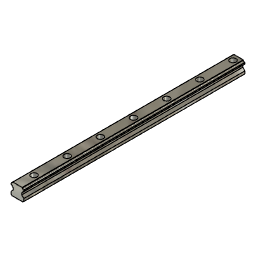
HGR25R_400 (Autodesk Fusion 360 design; units mm, degrees)
Autodesk Fusion 360 part; units mm, degrees
sketch "Sketch2" plane through (0, 0, 0) normal (0, 1, 0) x (1, 0, 0)
  line L0 (0, 0) -> (-10, 0)
  line L1 (-10, 0) -> (-11.5, -1.5)
  line L2 (-11.5, -1.5) -> (-11.5, -6.199)
  line L3 (-11.5, -6.199) -> (-7.7, -9.999)
  line L4 (-7.7, -9.999) -> (-7.7, -13.38)
  line L5 (-11.5, -17.08) -> (-11.5, -19.109)
  line L6 (-8.5085, -22) -> (0, -22)
  line L7 (0, -37) -> (0, 7) construction
  arc A0 (-8.9292, -21.5934) -> (-11.2845, -19.3172) centre (-11.447, -21.842) ccw
  line L8 (-11.5, -19.109) -> (-11.2845, -19.3172)
  line L9 (-8.9292, -21.5934) -> (-8.5085, -22)
  arc A1 (-11.2972, -16.8826) -> (-8.9263, -14.5741) centre (-11.447, -14.357) ccw
  line L10 (-7.7, -13.38) -> (-8.9263, -14.5741)
  line L11 (-11.2972, -16.8826) -> (-11.5, -17.08)
  line L12 (0, 0) -> (10, 0)
  line L13 (10, 0) -> (11.5, -1.5)
  line L14 (11.5, -1.5) -> (11.5, -6.199)
  line L15 (11.5, -6.199) -> (7.7, -9.999)
  line L16 (7.7, -9.999) -> (7.7, -13.38)
  line L17 (7.7, -13.38) -> (8.9263, -14.5741)
  arc A2 (8.9263, -14.5741) -> (11.2972, -16.8826) centre (11.447, -14.357) ccw
  line L18 (11.2972, -16.8826) -> (11.5, -17.08)
  line L19 (11.5, -17.08) -> (11.5, -19.109)
  line L20 (11.5, -19.109) -> (11.2845, -19.3172)
  arc A3 (11.2845, -19.3172) -> (8.9292, -21.5934) centre (11.447, -21.842) ccw
  line L21 (8.9292, -21.5934) -> (8.5085, -22)
  line L22 (8.5085, -22) -> (0, -22)
  dimension "d29" = 10
  dimension "d30" = 1.5
  dimension "d31" = 1.5
  dimension "d32" = 3.381
  dimension "d33" = 3.7
  dimension "d34" = 22
  dimension "d35" = 3.8
  dimension "d36" = 3.8
  dimension "d38" = 8.5085
  dimension "d39" = 2.029
  dimension "d40" = 2.891
  dimension "d42" = 11.447
  dimension "d43" = 0.158
  dimension "d46" = 2.53
  dimension "d47" = 2.53
  dimension "d48" = 7.485
  constraint coincident L0.start L12.start
  constraint horizontal L0
  constraint perpendicular L0 L2
  constraint perpendicular L0 L4
  constraint perpendicular L0 L5
  constraint perpendicular L5 L6
  constraint vertical L7
  constraint collinear L2 L5
  constraint coincident L0.start L7
  constraint coincident L6.end L7
  constraint coincident A0.start L8
  constraint collinear L8 L9
  constraint coincident A1.start L10
  constraint collinear L10 L11
  constraint vertical A0.centre A1.centre
  constraint symmetric L0.start L7 L12.start
  constraint symmetric L0.end L7 L12.end
  constraint symmetric L1.end L7 L13.end
  constraint symmetric L2.end L7 L14.end
  constraint symmetric L3.end L7 L15.end
  constraint symmetric L4.end L7 L16.end
  constraint symmetric L5.start L7 L18.end
  constraint symmetric L5.end L7 L19.end
  constraint symmetric L6.start L7 L21.end
  constraint symmetric L6.end L7 L22.end
  constraint symmetric L7 A0.end L20.end
  constraint symmetric L7 A0.start A3.end
  constraint symmetric L7 A0 A3
  constraint symmetric L7 A1.end L17.end
  constraint symmetric L7 A1.start A2.end
  constraint symmetric L7 A1 A2
  measures "d29" distance of L0.start L0.end
  measures "d30" vertical distance of L0.start L1.end
  measures "d31" distance of L0.end L2
  measures "d32" distance of L3.end L4.end
  measures "d33" vertical distance of L4.end L5.start
  measures "d34" distance of L0.start L6
  measures "d35" vertical distance of L2.end L3.end
  measures "d36" horizontal distance of L2.end L3.end
  measures "d38" distance of L6.start L7
  measures "d39" distance of L5.start L5.end
  measures "d40" distance of L5.end L6
  measures "d42" distance of L7 A0.centre
  measures "d43" distance of L6 A0.centre
  measures "d46" radius of A0
  measures "d47" radius of A1
  measures "d48" distance of A0.centre A1.centre
extrude "Extrude2" add sketch "Sketch2" along normal blind 400
hole "Hole4" at (0, 30, 22) direction (0, 0, -1) diameter 7 end up to surface (22 mm away) counterbore diameter 11 counterbore depth 9
pattern_linear "R-Pattern4" count 7 spacing 60 along (0, 1, 0) of "Hole4"
equation "RailLength = 400 mm"
equation "RailHoleSpacing = 60 mm"
equation "RailFirstHoleOffset = ( RailLength - ( ( RailNumberOfHoles - 1 ) * RailHoleSpacing ) ) / 2"
equation "d53 = RailLength"
equation "RailNumberOfHoles = round(RailLength / RailHoleSpacing)"
equation "d94 = RailNumberOfHoles"
equation "d96 = RailHoleSpacing"
